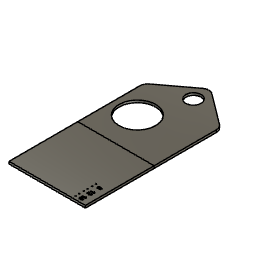
Lid (Autodesk Fusion 360 design; units mm, degrees)
Autodesk Fusion 360 part; units mm, degrees
sketch "Sketch1" plane through (0, 0, 0) normal (0, 0, 1) x (1, 0, 0)
  line L0 (0, 0) -> (100, 0)
  line L1 (100, 0) -> (100, 171.5)
  line L2 (100, 171.5) -> (0, 171.5)
  line L3 (0, 171.5) -> (0, 0)
  line L4 (56, 209.5) -> (96, 179.5)
  line L5 (4, 179.5) -> (44, 209.5)
  arc A0 (56, 209.5) -> (44, 209.5) centre (50, 201.5) ccw
  arc A1 (100, 171.5) -> (96, 179.5) centre (90, 171.5) ccw
  arc A2 (4, 179.5) -> (0, 171.5) centre (10, 171.5) ccw
  circle A3 centre (50, 191.5) radius 10
  dimension "d1" = 100
  dimension "d2" = 171.5
  dimension "d3" = 20
  dimension "d4" = 20
  dimension "d5" = 20
  dimension "d6" = 30
  dimension "d7" = 50
  dimension "d8" = 50
  dimension "d9" = 50
  dimension "d10" = 20
  dimension "d11" = 20
  dimension "d12" = 50
  constraint horizontal L0
  constraint vertical L1
  constraint horizontal L2
  constraint vertical L3
  constraint coincident L0.start L3.end
  constraint coincident L2 A2.centre
  constraint coincident L2 A1.centre
  constraint tangent L4 A1
  constraint tangent L5 A0
  measures "d1" distance of L0.start L0.end
  measures "d2" distance of L0.start L2.end
  measures "d3" diameter of A2
  measures "d4" diameter of A1
  measures "d5" diameter of A0
  measures "d6" distance of L2 A0.centre
  measures "d7" distance of L3 A0.centre
  measures "d8" distance of L5.start L5.end
  measures "d9" distance of L4.start L4.end
  measures "d10" diameter of A3
  measures "d11" distance of L2 A3.centre
  measures "d12" horizontal distance of L2.end A3.centre
extrude "Extrude1" add sketch "Sketch1" along normal blind 3 makes body 1
sketch "Sketch2" plane through (0, 0, 3) normal (0, 0, 1) x (-1, 0, 0)
  circle A0 centre (-50, -191.5) radius 10
  arc A1 (-56, -209.5) -> (-44, -209.5) centre (-50, -201.5) ccw
  line L0 (-44, -209.5) -> (-4, -179.5)
  arc A2 (-4, -179.5) -> (0, -171.5) centre (-10, -171.5) ccw
  line L1 (0, -171.5) -> (0, 0)
  line L2 (0, 0) -> (-100, 0)
  line L3 (-100, 0) -> (-100, -171.5)
  arc A3 (-100, -171.5) -> (-96, -179.5) centre (-90, -171.5) ccw
  line L4 (-96, -179.5) -> (-56, -209.5)
  line L5 (0, 0) -> (-100, 0) construction
  line L6 (-100, 0) -> (-100, -171.5) construction
  line L7 (-100, -171.5) -> (0, -171.5) construction
  line L8 (0, -171.5) -> (0, 0) construction
  circle A4 centre (-31.5, -136.5) radius 24
  dimension "d15" = 171.5
  dimension "d16" = 100
  dimension "d17" = 48
  dimension "d18" = 31.5
  dimension "d19" = 35
  constraint horizontal L5
  constraint vertical L6
  constraint horizontal L7
  constraint vertical L8
  constraint coincident L1.end L2.start
  measures "d15" distance of L1.end A2.end
  measures "d16" distance of L1.end L2.end
  measures "d17" diameter of A4
  measures "d18" distance of L8 A4.centre
  measures "d19" distance of L7 A4.centre
extrude "Extrude2" cut sketch "Sketch2" against normal blind 3 contours A4 bodies 1
sketch "Sketch3" plane through (0, 0, 3) normal (0, 0, 1) x (-1, 0, 0)
  circle A0 centre (-31.5, -136.5) radius 24
  circle A1 centre (-50, -191.5) radius 10
  arc A2 (-56, -209.5) -> (-44, -209.5) centre (-50, -201.5) ccw
  line L0 (-44, -209.5) -> (-4, -179.5)
  arc A3 (-4, -179.5) -> (0, -171.5) centre (-10, -171.5) ccw
  line L1 (0, -171.5) -> (0, 0)
  line L2 (0, 0) -> (-100, 0)
  line L3 (-100, 0) -> (-100, -171.5)
  arc A4 (-100, -171.5) -> (-96, -179.5) centre (-90, -171.5) ccw
  line L4 (-96, -179.5) -> (-56, -209.5)
  line L5 (-95, -65) -> (-95, 0) construction
  line L6 (-82, -5) -> (-83, -5)
  line L7 (-83, -5) -> (-83, -4)
  line L8 (-83, -4) -> (-82, -4)
  line L9 (-82, -4) -> (-82, -5)
  line L10 (-82, -10) -> (-83, -10)
  line L11 (-83, -10) -> (-83, -9)
  line L12 (-83, -9) -> (-82, -9)
  line L13 (-82, -9) -> (-82, -10)
  line L14 (-82, -16) -> (-83, -16)
  line L15 (-83, -16) -> (-83, -15)
  line L16 (-83, -15) -> (-82, -15)
  line L17 (-82, -15) -> (-82, -16)
  line L18 (-82, -21) -> (-83, -21)
  line L19 (-83, -21) -> (-83, -20)
  line L20 (-83, -20) -> (-82, -20)
  line L21 (-82, -20) -> (-82, -21)
  line L22 (-82, -27) -> (-83, -27)
  line L23 (-83, -27) -> (-83, -26)
  line L24 (-83, -26) -> (-82, -26)
  line L25 (-82, -26) -> (-82, -27)
  line L26 (-82, -32) -> (-83, -32)
  line L27 (-83, -32) -> (-83, -31)
  line L28 (-83, -31) -> (-82, -31)
  line L29 (-82, -31) -> (-82, -32)
  line L30 (-86, -35) -> (-86, 0) construction
  line L31 (-87, -32) -> (-87, -26) construction
  line L32 (-87, -26) -> (-92, -26) construction
  line L33 (-92, -26) -> (-92, -32) construction
  line L34 (-92, -32) -> (-87, -32) construction
  line L35 (-87, -21) -> (-87, -15) construction
  line L36 (-87, -15) -> (-92, -15) construction
  line L37 (-92, -15) -> (-92, -21) construction
  line L38 (-92, -21) -> (-87, -21) construction
  line L39 (-87, -10) -> (-87, -4) construction
  line L40 (-87, -4) -> (-92, -4) construction
  line L41 (-92, -4) -> (-92, -10) construction
  line L42 (-92, -10) -> (-87, -10) construction
  dimension "d22" = 5
  dimension "d23" = 1
  dimension "d24" = 1
  dimension "d25" = 1
  dimension "d26" = 1
  dimension "d27" = 1
  dimension "d28" = 1
  dimension "d29" = 1
  dimension "d30" = 1
  dimension "d31" = 1
  dimension "d32" = 1
  dimension "d33" = 1
  dimension "d34" = 1
  dimension "d36" = 5
  dimension "d37" = 6
  dimension "d38" = 6
  dimension "d39" = 5
  dimension "d40" = 6
  dimension "d41" = 5
  dimension "d42" = 5
  dimension "d43" = 5
  text T0 "8" font "Arial" height 5 bold align centre middle in box 6 x 5 at (-87, -32) x (0, 1) y (-1, 0) spacing 1 kerned
  text T1 "12" font "Arial" height 5 bold align centre middle in box 6 x 5 at (-87, -21) x (0, 1) y (-1, 0) spacing 1 kerned
  text T2 "16" font "Arial" height 5 bold align centre middle in box 6 x 5 at (-87, -10) x (0, 1) y (-1, 0) spacing 1 kerned
  constraint coincident L2 L5.end
  constraint perpendicular L2 L5
  constraint horizontal L6
  constraint vertical L7
  constraint horizontal L8
  constraint vertical L9
  constraint horizontal L10
  constraint vertical L11
  constraint horizontal L12
  constraint vertical L13
  constraint horizontal L14
  constraint vertical L15
  constraint horizontal L16
  constraint vertical L17
  constraint horizontal L18
  constraint vertical L19
  constraint horizontal L20
  constraint vertical L21
  constraint horizontal L22
  constraint vertical L23
  constraint horizontal L24
  constraint vertical L25
  constraint horizontal L26
  constraint vertical L27
  constraint horizontal L28
  constraint vertical L29
  constraint coincident L2 L30.end
  constraint perpendicular L2 L30
  measures "d22" distance of L3 L5
  measures "d23" distance of L10.end L11.end
  measures "d24" distance of L6.end L7.end
  measures "d25" distance of L14.end L15.end
  measures "d26" distance of L18.end L19.end
  measures "d27" distance of L22.end L23.end
  measures "d28" distance of L26.end L27.end
  measures "d29" distance of L26.start L26.end
  measures "d30" distance of L22.start L22.end
  measures "d31" distance of L18.start L18.end
  measures "d32" distance of L14.start L14.end
  measures "d33" distance of L10.start L10.end
  measures "d34" distance of L6.start L6.end
  measures "d36" distance of L18 L24
  measures "d37" distance of L24 L26
  measures "d38" distance of L16 L18
  measures "d39" distance of L10 L16
  measures "d40" distance of L8 L10
extrude "Extrude3" cut sketch "Sketch3" against normal blind 2 text T0 T1 T2 bodies 1
extrude "Extrude4" cut sketch "Sketch3" against normal blind 3 contours L6 L7 L8 L9 | L10 L11 L12 L13 | L14 L15 L16 L17 | L18 L19 L20 L21 | L22 L23 L24 L25 | L26 L27 L28 L29 bodies 1
sketch "Sketch4" plane through (0, 0, 3) normal (0, 0, 1) x (-1, 0, 0)
  line L0 (-83, -16) -> (-83, -15)
  line L1 (-83, -15) -> (-82, -15)
  line L2 (-82, -15) -> (-82, -16)
  line L3 (-82, -16) -> (-83, -16)
  line L4 (-83, -32) -> (-83, -31)
  line L5 (-83, -31) -> (-82, -31)
  line L6 (-82, -31) -> (-82, -32)
  line L7 (-82, -32) -> (-83, -32)
  line L8 (-83, -10) -> (-83, -9)
  line L9 (-83, -9) -> (-82, -9)
  line L10 (-82, -9) -> (-82, -10)
  line L11 (-82, -10) -> (-83, -10)
  line L12 (-83, -21) -> (-83, -20)
  line L13 (-83, -20) -> (-82, -20)
  line L14 (-82, -20) -> (-82, -21)
  line L15 (-82, -21) -> (-83, -21)
  line L16 (-83, -27) -> (-83, -26)
  line L17 (-83, -26) -> (-82, -26)
  line L18 (-82, -26) -> (-82, -27)
  line L19 (-82, -27) -> (-83, -27)
  line L20 (-83, -5) -> (-83, -4)
  line L21 (-83, -4) -> (-82, -4)
  line L22 (-82, -4) -> (-82, -5)
  line L23 (-82, -5) -> (-83, -5)
  arc A0 (-56, -209.5) -> (-44, -209.5) centre (-50, -201.5) ccw
  line L24 (-44, -209.5) -> (-4, -179.5)
  arc A1 (-4, -179.5) -> (0, -171.5) centre (-10, -171.5) ccw
  line L25 (0, -171.5) -> (0, 0)
  line L26 (0, 0) -> (-100, 0)
  line L27 (-100, 0) -> (-100, -171.5)
  arc A2 (-100, -171.5) -> (-96, -179.5) centre (-90, -171.5) ccw
  line L28 (-96, -179.5) -> (-56, -209.5)
  circle A3 centre (-50, -191.5) radius 10
  circle A4 centre (-31.5, -136.5) radius 24
  line L29 (-92.0205, -9.0651) -> (-92.0205, -8.2875)
  line L30 (-92.0205, -8.2875) -> (-87, -8.2875)
  line L31 (-87, -8.2875) -> (-87, -9.2459)
  line L32 (-87, -9.2459) -> (-90.6119, -9.2459)
  spline S0 degree 3 poles (-90.6119, -9.2459) (-90.4584, -9.4301) (-90.148, -9.8026) (-89.9736, -10.2552) (-89.8854, -10.484) knots 0 0 0 0 0.071402 0.144411 0.144411 0.144411 0.144411
  line L33 (-89.8854, -10.484) -> (-90.7551, -10.484)
  spline S1 degree 3 poles (-90.7551, -10.484) (-90.8095, -10.3508) (-90.9288, -10.0589) (-91.1179, -9.8062) (-91.2207, -9.6688) knots 0 0 0 0 0.042986 0.09421 0.09421 0.09421 0.09421
  spline S2 degree 3 poles (-91.2207, -9.6688) (-91.3367, -9.5348) (-91.5605, -9.2762) (-91.8709, -9.1338) (-92.0205, -9.0651) knots 0 0 0 0 0.052484 0.101245 0.101245 0.101245 0.101245
  line L34 (-92.0205, -20.014) -> (-92.0205, -19.2364)
  line L35 (-92.0205, -19.2364) -> (-87, -19.2364)
  line L36 (-87, -19.2364) -> (-87, -20.1947)
  line L37 (-87, -20.1947) -> (-90.6119, -20.1947)
  spline S3 degree 3 poles (-90.6119, -20.1947) (-90.4584, -20.3789) (-90.148, -20.7515) (-89.9736, -21.204) (-89.8854, -21.4328) knots 0 0 0 0 0.071402 0.144411 0.144411 0.144411 0.144411
  line L38 (-89.8854, -21.4328) -> (-90.7551, -21.4328)
  spline S4 degree 3 poles (-90.7551, -21.4328) (-90.8095, -21.2996) (-90.9288, -21.0078) (-91.1179, -20.7551) (-91.2207, -20.6177) knots 0 0 0 0 0.042986 0.09421 0.09421 0.09421 0.09421
  spline S5 degree 3 poles (-91.2207, -20.6177) (-91.3367, -20.4836) (-91.5605, -20.2251) (-91.8709, -20.0826) (-92.0205, -20.014) knots 0 0 0 0 0.052484 0.101245 0.101245 0.101245 0.101245
  spline S6 degree 3 poles (-88.4291, -30.6439) (-88.5611, -30.6358) (-88.8234, -30.6197) (-89.0579, -30.5014) (-89.1743, -30.4427) knots 0 0 0 0 0.039248 0.077913 0.077913 0.077913 0.077913
  spline S7 degree 3 poles (-89.1743, -30.4427) (-89.2822, -30.3628) (-89.5089, -30.1951) (-89.6329, -29.9412) (-89.6978, -29.8083) knots 0 0 0 0 0.03969 0.083332 0.083332 0.083332 0.083332
  spline S8 degree 3 poles (-89.6978, -29.8083) (-89.752, -29.9218) (-89.8541, -30.1359) (-90.0413, -30.2808) (-90.1293, -30.3489) knots 0 0 0 0 0.037117 0.070026 0.070026 0.070026 0.070026
  spline S9 degree 3 poles (-90.1293, -30.3489) (-90.2232, -30.3982) (-90.4119, -30.497) (-90.6245, -30.5108) (-90.7312, -30.5177) knots 0 0 0 0 0.03144 0.063142 0.063142 0.063142 0.063142
  spline S10 degree 3 poles (-90.7312, -30.5177) (-90.9088, -30.5023) (-91.2593, -30.4719) (-91.5246, -30.2411) (-91.6555, -30.1272) knots 0 0 0 0 0.051999 0.102674 0.102674 0.102674 0.102674
  spline S11 degree 3 poles (-91.6555, -30.1272) (-91.7618, -29.9748) (-91.9933, -29.6428) (-92.0109, -29.2367) (-92.0205, -29.0171) knots 0 0 0 0 0.054631 0.119017 0.119017 0.119017 0.119017
  spline S12 degree 3 poles (-92.0205, -29.0171) (-92.0106, -28.7989) (-91.9923, -28.3942) (-91.7618, -28.063) (-91.6555, -27.9103) knots 0 0 0 0 0.063964 0.118669 0.118669 0.118669 0.118669
  spline S13 degree 3 poles (-91.6555, -27.9103) (-91.5247, -27.7954) (-91.26, -27.5629) (-90.9089, -27.532) (-90.7312, -27.5164) knots 0 0 0 0 0.050824 0.102839 0.102839 0.102839 0.102839
  spline S14 degree 3 poles (-90.7312, -27.5164) (-90.6193, -27.5234) (-90.3992, -27.5371) (-90.2068, -27.6444) (-90.1122, -27.6971) knots 0 0 0 0 0.033179 0.065222 0.065222 0.065222 0.065222
  spline S15 degree 3 poles (-90.1122, -27.6971) (-90.0266, -27.7648) (-89.8511, -27.9035) (-89.7497, -28.1031) (-89.6978, -28.2053) knots 0 0 0 0 0.032323 0.06627 0.06627 0.06627 0.06627
  spline S16 degree 3 poles (-89.6978, -28.2053) (-89.638, -28.0765) (-89.5228, -27.8286) (-89.3116, -27.6557) (-89.2101, -27.5726) knots 0 0 0 0 0.041993 0.080807 0.080807 0.080807 0.080807
  spline S17 degree 3 poles (-89.2101, -27.5726) (-89.0977, -27.5095) (-88.8678, -27.3804) (-88.6045, -27.3643) (-88.47, -27.3561) knots 0 0 0 0 0.038162 0.07801 0.07801 0.07801 0.07801
  spline S18 degree 3 poles (-88.47, -27.3561) (-88.2525, -27.372) (-87.8308, -27.403) (-87.5031, -27.669) (-87.3445, -27.7977) knots 0 0 0 0 0.06372 0.123527 0.123527 0.123527 0.123527
  spline S19 degree 3 poles (-87.3445, -27.7977) (-87.2182, -27.9625) (-86.9531, -28.3083) (-86.9257, -28.7443) (-86.9113, -28.9727) knots 0 0 0 0 0.060855 0.127775 0.127775 0.127775 0.127775
  spline S20 degree 3 poles (-86.9113, -28.9727) (-86.9234, -29.1868) (-86.9464, -29.5966) (-87.165, -29.943) (-87.2694, -30.1085) knots 0 0 0 0 0.063138 0.120844 0.120844 0.120844 0.120844
  spline S21 degree 3 poles (-87.2694, -30.1085) (-87.4261, -30.2646) (-87.7466, -30.5841) (-88.1982, -30.6237) (-88.4291, -30.6439) knots 0 0 0 0 0.064238 0.131411 0.131411 0.131411 0.131411
  spline S22 degree 3 poles (-88.1562, -16.2742) (-88.1122, -16.312) (-88.0283, -16.3839) (-87.9347, -16.4425) (-87.8902, -16.4703) knots 0 0 0 0 0.017365 0.033092 0.033092 0.033092 0.033092
  line L39 (-87.8902, -16.4703) -> (-87.8902, -14.5672)
  line L40 (-87.8902, -14.5672) -> (-87, -14.5672)
  line L41 (-87, -14.5672) -> (-87, -17.9267)
  spline S23 degree 3 poles (-87, -17.9267) (-87.1668, -17.8989) (-87.5038, -17.8429) (-87.8047, -17.681) (-87.9567, -17.5992) knots 0 0 0 0 0.050353 0.101733 0.101733 0.101733 0.101733
  spline S24 degree 3 poles (-87.9567, -17.5992) (-88.1357, -17.4683) (-88.5712, -17.1498) (-88.939, -16.7543) (-89.1555, -16.5215) knots 0 0 0 0 0.066412 0.161523 0.161523 0.161523 0.161523
  spline S25 degree 3 poles (-89.1555, -16.5215) (-89.3199, -16.3425) (-89.5777, -16.0618) (-89.8686, -15.8159) (-89.9741, -15.7268) knots 0 0 0 0 0.072782 0.114179 0.114179 0.114179 0.114179
  spline S26 degree 3 poles (-89.9741, -15.7268) (-90.0697, -15.6692) (-90.2511, -15.5599) (-90.4614, -15.5389) (-90.5607, -15.529) knots 0 0 0 0 0.033023 0.0626 0.0626 0.0626 0.0626
  spline S27 degree 3 poles (-90.5607, -15.529) (-90.6588, -15.5337) (-90.8409, -15.5424) (-90.9864, -15.6511) (-91.0535, -15.7012) knots 0 0 0 0 0.028676 0.053274 0.053274 0.053274 0.053274
  spline S28 degree 3 poles (-91.0535, -15.7012) (-91.1037, -15.7669) (-91.2107, -15.9069) (-91.2205, -16.0833) (-91.2258, -16.177) knots 0 0 0 0 0.024236 0.051648 0.051648 0.051648 0.051648
  spline S29 degree 3 poles (-91.2258, -16.177) (-91.2198, -16.2704) (-91.2084, -16.4486) (-91.0977, -16.5881) (-91.045, -16.6545) knots 0 0 0 0 0.02732 0.052153 0.052153 0.052153 0.052153
  spline S30 degree 3 poles (-91.045, -16.6545) (-90.9673, -16.7076) (-90.7873, -16.8306) (-90.5688, -16.8488) (-90.4447, -16.8591) knots 0 0 0 0 0.027816 0.064377 0.064377 0.064377 0.064377
  line L42 (-90.4447, -16.8591) -> (-90.5402, -17.8141)
  spline S31 degree 3 poles (-90.5402, -17.8141) (-90.7784, -17.7788) (-91.2135, -17.7143) (-91.5319, -17.4144) (-91.676, -17.2786) knots 0 0 0 0 0.070212 0.128259 0.128259 0.128259 0.128259
  spline S32 degree 3 poles (-91.676, -17.2786) (-91.7764, -17.1143) (-91.9872, -16.7694) (-92.009, -16.3649) (-92.0205, -16.1531) knots 0 0 0 0 0.056857 0.119356 0.119356 0.119356 0.119356
  spline S33 degree 3 poles (-92.0205, -16.1531) (-92.0088, -15.9252) (-91.9868, -15.4977) (-91.7377, -15.1516) (-91.6214, -14.9901) knots 0 0 0 0 0.06683 0.125293 0.125293 0.125293 0.125293
  spline S34 degree 3 poles (-91.6214, -14.9901) (-91.4797, -14.8668) (-91.1947, -14.6186) (-90.8183, -14.5844) (-90.6289, -14.5672) knots 0 0 0 0 0.054863 0.110365 0.110365 0.110365 0.110365
  spline S35 degree 3 poles (-90.6289, -14.5672) (-90.5181, -14.5721) (-90.298, -14.5818) (-90.0895, -14.653) (-89.986, -14.6883) knots 0 0 0 0 0.033094 0.065719 0.065719 0.065719 0.065719
  spline S36 degree 3 poles (-89.986, -14.6883) (-89.8799, -14.7371) (-89.6528, -14.8415) (-89.4529, -14.9919) (-89.3465, -15.072) knots 0 0 0 0 0.034948 0.074768 0.074768 0.074768 0.074768
  spline S37 degree 3 poles (-89.3465, -15.072) (-89.2552, -15.152) (-89.0305, -15.3487) (-88.8286, -15.5689) (-88.7087, -15.6995) knots 0 0 0 0 0.036404 0.089534 0.089534 0.089534 0.089534
  spline S38 degree 3 poles (-88.7087, -15.6995) (-88.5948, -15.8245) (-88.4158, -16.021) (-88.2255, -16.2066) (-88.1562, -16.2742) knots 0 0 0 0 0.050705 0.079736 0.079736 0.079736 0.079736
  spline S39 degree 3 poles (-92.0205, -5.0269) (-92.0095, -4.848) (-91.9884, -4.5042) (-91.7945, -4.2201) (-91.7016, -4.0839) knots 0 0 0 0 0.052662 0.101211 0.101211 0.101211 0.101211
  spline S40 degree 3 poles (-91.7016, -4.0839) (-91.5777, -3.9699) (-91.3136, -3.7268) (-90.9621, -3.6493) (-90.7756, -3.6081) knots 0 0 0 0 0.049626 0.10577 0.10577 0.10577 0.10577
  line L43 (-90.7756, -3.6081) -> (-90.6733, -4.5358)
  spline S41 degree 3 poles (-90.6733, -4.5358) (-90.7595, -4.5489) (-90.9161, -4.5725) (-91.0404, -4.6696) (-91.0962, -4.7132) knots 0 0 0 0 0.025643 0.046549 0.046549 0.046549 0.046549
  spline S42 degree 3 poles (-91.0962, -4.7132) (-91.136, -4.7659) (-91.2188, -4.8757) (-91.2279, -5.0134) (-91.2326, -5.0849) knots 0 0 0 0 0.019378 0.040376 0.040376 0.040376 0.040376
  spline S43 degree 3 poles (-91.2326, -5.0849) (-91.2197, -5.1834) (-91.1928, -5.3878) (-91.0393, -5.5264) (-90.9598, -5.5982) knots 0 0 0 0 0.028828 0.059854 0.059854 0.059854 0.059854
  spline S44 degree 3 poles (-90.9598, -5.5982) (-90.8215, -5.6624) (-90.4636, -5.8287) (-90.0673, -5.8497) (-89.824, -5.8626) knots 0 0 0 0 0.04538 0.117524 0.117524 0.117524 0.117524
  spline S45 degree 3 poles (-89.824, -5.8626) (-89.9474, -5.737) (-90.1912, -5.4888) (-90.2285, -5.1432) (-90.2469, -4.9724) knots 0 0 0 0 0.051176 0.101164 0.101164 0.101164 0.101164
  spline S46 degree 3 poles (-90.2469, -4.9724) (-90.227, -4.7786) (-90.1866, -4.3864) (-89.9232, -4.0927) (-89.7899, -3.9441) knots 0 0 0 0 0.056881 0.115141 0.115141 0.115141 0.115141
  spline S47 degree 3 poles (-89.7899, -3.9441) (-89.622, -3.8193) (-89.2722, -3.5593) (-88.8364, -3.5308) (-88.6098, -3.516) knots 0 0 0 0 0.061412 0.127933 0.127933 0.127933 0.127933
  spline S48 degree 3 poles (-88.6098, -3.516) (-88.3708, -3.5309) (-87.9146, -3.5594) (-87.5515, -3.835) (-87.3786, -3.9662) knots 0 0 0 0 0.070061 0.133726 0.133726 0.133726 0.133726
  spline S49 degree 3 poles (-87.3786, -3.9662) (-87.2433, -4.1298) (-86.9659, -4.4651) (-86.9321, -4.8997) (-86.9147, -5.1224) knots 0 0 0 0 0.062079 0.127323 0.127323 0.127323 0.127323
  spline S50 degree 3 poles (-86.9147, -5.1224) (-86.9395, -5.3638) (-86.9892, -5.8479) (-87.3315, -6.1939) (-87.5031, -6.3673) knots 0 0 0 0 0.070531 0.141441 0.141441 0.141441 0.141441
  spline S51 degree 3 poles (-87.5031, -6.3673) (-87.7564, -6.5088) (-88.3517, -6.8413) (-89.0377, -6.85) (-89.4318, -6.855) knots 0 0 0 0 0.085821 0.201701 0.201701 0.201701 0.201701
  spline S52 degree 3 poles (-89.4318, -6.855) (-89.8364, -6.8495) (-90.5422, -6.8398) (-91.1528, -6.4943) (-91.4134, -6.3469) knots 0 0 0 0 0.118944 0.207464 0.207464 0.207464 0.207464
  spline S53 degree 3 poles (-91.4134, -6.3469) (-91.5904, -6.1639) (-91.9471, -5.7952) (-91.9959, -5.2843) (-92.0205, -5.0269) knots 0 0 0 0 0.074058 0.149191 0.149191 0.149191 0.149191
sketch "Sketch5" plane through (0, 0, 3) normal (0, 0, 1) x (-1, 0, 0)
  line L0 (-68, -32) -> (-67, -32)
  line L1 (-67, -32) -> (-67, -31)
  line L2 (-67, -31) -> (-68, -31)
  line L3 (-68, -31) -> (-68, -32)
  line L4 (-68, -27) -> (-67, -27)
  line L5 (-67, -27) -> (-67, -26)
  line L6 (-67, -26) -> (-68, -26)
  line L7 (-68, -26) -> (-68, -27)
  line L8 (-68, -21) -> (-67, -21)
  line L9 (-67, -21) -> (-67, -20)
  line L10 (-67, -20) -> (-68, -20)
  line L11 (-68, -20) -> (-68, -21)
  line L12 (-68, -16) -> (-67, -16)
  line L13 (-67, -16) -> (-67, -15)
  line L14 (-67, -15) -> (-68, -15)
  line L15 (-68, -15) -> (-68, -16)
  line L16 (-68, -10) -> (-67, -10)
  line L17 (-67, -10) -> (-67, -9)
  line L18 (-67, -9) -> (-68, -9)
  line L19 (-68, -9) -> (-68, -10)
  line L20 (-68, -5) -> (-67, -5)
  line L21 (-67, -5) -> (-67, -4)
  line L22 (-67, -4) -> (-68, -4)
  line L23 (-68, -4) -> (-68, -5)
  constraint horizontal L0
  constraint vertical L1
  constraint horizontal L2
  constraint vertical L3
  constraint horizontal L4
  constraint vertical L5
  constraint horizontal L6
  constraint vertical L7
  constraint horizontal L8
  constraint vertical L9
  constraint horizontal L10
  constraint vertical L11
  constraint horizontal L12
  constraint vertical L13
  constraint horizontal L14
  constraint vertical L15
  constraint horizontal L16
  constraint vertical L17
  constraint horizontal L18
  constraint vertical L19
  constraint horizontal L20
  constraint vertical L21
  constraint horizontal L22
  constraint vertical L23
extrude "Extrude5" cut sketch "Sketch5" against normal blind 3 bodies 1
sketch "Sketch6" plane through (0, 0, 3) normal (0, 0, 1) x (-1, 0, 0)
  line L0 (-71, -32) -> (-71, 0) construction
  line L1 (-72, -32) -> (-72, -26) construction
  line L2 (-72, -26) -> (-78, -26) construction
  line L3 (-78, -26) -> (-78, -32) construction
  line L4 (-78, -32) -> (-72, -32) construction
  line L5 (-72, -21) -> (-72, -15) construction
  line L6 (-72, -15) -> (-78, -15) construction
  line L7 (-78, -15) -> (-78, -21) construction
  line L8 (-78, -21) -> (-72, -21) construction
  line L9 (-72, -10) -> (-72, -4) construction
  line L10 (-72, -4) -> (-78, -4) construction
  line L11 (-78, -4) -> (-78, -10) construction
  line L12 (-78, -10) -> (-72, -10) construction
  dimension "d50" = 5
  dimension "d51" = 5
  dimension "d52" = 5
  text T0 "H" font "Arial" height 5 bold align centre middle in box 6 x 6 at (-72, -32) x (0, 1) y (-1, 0) spacing 1 kerned
  text T1 "M" font "Arial" height 5 bold align centre middle in box 6 x 6 at (-72, -21) x (0, 1) y (-1, 0) spacing 1 kerned
  text T2 "L" font "Arial" height 5 bold align centre middle in box 6 x 6 at (-72, -10) x (0, 1) y (-1, 0) spacing 1 kerned
  constraint vertical L0
extrude "Extrude6" cut sketch "Sketch6" against normal blind 2 text T0 T1 T2 bodies 1
ref_plane "WorkPlane1" through (0, 90, 0) normal (0, 1, 0) x (0, 0, 1)
split "Split1" by plane through (0, 90, 0) normal (0, 1, 0) bodies 1 makes body 2 at (85.0773, 131.4743, 0)
sketch "Sketch8" plane through (0, 0, 3) normal (0, 0, 1) x (-1, 0, 0)
  spline S0 degree 3 poles (-92.0205, -5.0269) (-92.0095, -4.848) (-91.9884, -4.5042) (-91.7945, -4.2201) (-91.7016, -4.0839) knots 0 0 0 0 0.052662 0.101211 0.101211 0.101211 0.101211
  spline S1 degree 3 poles (-91.7016, -4.0839) (-91.5777, -3.9699) (-91.3136, -3.7268) (-90.9621, -3.6493) (-90.7756, -3.6081) knots 0 0 0 0 0.049626 0.10577 0.10577 0.10577 0.10577
  line L0 (-90.7756, -3.6081) -> (-90.6733, -4.5358)
  spline S2 degree 3 poles (-90.6733, -4.5358) (-90.7595, -4.5489) (-90.9161, -4.5725) (-91.0404, -4.6696) (-91.0962, -4.7132) knots 0 0 0 0 0.025643 0.046549 0.046549 0.046549 0.046549
  spline S3 degree 3 poles (-91.0962, -4.7132) (-91.136, -4.7659) (-91.2188, -4.8757) (-91.2279, -5.0134) (-91.2326, -5.0849) knots 0 0 0 0 0.019378 0.040376 0.040376 0.040376 0.040376
  spline S4 degree 3 poles (-91.2326, -5.0849) (-91.2197, -5.1834) (-91.1928, -5.3878) (-91.0393, -5.5264) (-90.9598, -5.5982) knots 0 0 0 0 0.028828 0.059854 0.059854 0.059854 0.059854
  spline S5 degree 3 poles (-90.9598, -5.5982) (-90.8215, -5.6624) (-90.4636, -5.8287) (-90.0673, -5.8497) (-89.824, -5.8626) knots 0 0 0 0 0.04538 0.117524 0.117524 0.117524 0.117524
  spline S6 degree 3 poles (-89.824, -5.8626) (-89.9474, -5.737) (-90.1912, -5.4888) (-90.2285, -5.1432) (-90.2469, -4.9724) knots 0 0 0 0 0.051176 0.101164 0.101164 0.101164 0.101164
  spline S7 degree 3 poles (-90.2469, -4.9724) (-90.227, -4.7786) (-90.1866, -4.3864) (-89.9232, -4.0927) (-89.7899, -3.9441) knots 0 0 0 0 0.056881 0.115141 0.115141 0.115141 0.115141
  spline S8 degree 3 poles (-89.7899, -3.9441) (-89.622, -3.8193) (-89.2722, -3.5593) (-88.8364, -3.5308) (-88.6098, -3.516) knots 0 0 0 0 0.061412 0.127933 0.127933 0.127933 0.127933
  spline S9 degree 3 poles (-88.6098, -3.516) (-88.3708, -3.5309) (-87.9146, -3.5594) (-87.5515, -3.835) (-87.3786, -3.9662) knots 0 0 0 0 0.070061 0.133726 0.133726 0.133726 0.133726
  spline S10 degree 3 poles (-87.3786, -3.9662) (-87.2433, -4.1298) (-86.9659, -4.4651) (-86.9321, -4.8997) (-86.9147, -5.1224) knots 0 0 0 0 0.062079 0.127323 0.127323 0.127323 0.127323
  spline S11 degree 3 poles (-86.9147, -5.1224) (-86.9395, -5.3638) (-86.9892, -5.8479) (-87.3315, -6.1939) (-87.5031, -6.3673) knots 0 0 0 0 0.070531 0.141441 0.141441 0.141441 0.141441
  spline S12 degree 3 poles (-87.5031, -6.3673) (-87.7564, -6.5088) (-88.3517, -6.8413) (-89.0377, -6.85) (-89.4318, -6.855) knots 0 0 0 0 0.085821 0.201701 0.201701 0.201701 0.201701
  spline S13 degree 3 poles (-89.4318, -6.855) (-89.8364, -6.8495) (-90.5422, -6.8398) (-91.1528, -6.4943) (-91.4134, -6.3469) knots 0 0 0 0 0.118944 0.207464 0.207464 0.207464 0.207464
  spline S14 degree 3 poles (-91.4134, -6.3469) (-91.5904, -6.1639) (-91.9471, -5.7952) (-91.9959, -5.2843) (-92.0205, -5.0269) knots 0 0 0 0 0.074058 0.149191 0.149191 0.149191 0.149191
  spline S15 degree 3 poles (-88.1562, -16.2742) (-88.1122, -16.312) (-88.0283, -16.3839) (-87.9347, -16.4425) (-87.8902, -16.4703) knots 0 0 0 0 0.017365 0.033092 0.033092 0.033092 0.033092
  line L1 (-87.8902, -16.4703) -> (-87.8902, -14.5672)
  line L2 (-87.8902, -14.5672) -> (-87, -14.5672)
  line L3 (-87, -14.5672) -> (-87, -17.9267)
  spline S16 degree 3 poles (-87, -17.9267) (-87.1668, -17.8989) (-87.5038, -17.8429) (-87.8047, -17.681) (-87.9567, -17.5992) knots 0 0 0 0 0.050353 0.101733 0.101733 0.101733 0.101733
  spline S17 degree 3 poles (-87.9567, -17.5992) (-88.1357, -17.4683) (-88.5712, -17.1498) (-88.939, -16.7543) (-89.1555, -16.5215) knots 0 0 0 0 0.066412 0.161523 0.161523 0.161523 0.161523
  spline S18 degree 3 poles (-89.1555, -16.5215) (-89.3199, -16.3425) (-89.5777, -16.0618) (-89.8686, -15.8159) (-89.9741, -15.7268) knots 0 0 0 0 0.072782 0.114179 0.114179 0.114179 0.114179
  spline S19 degree 3 poles (-89.9741, -15.7268) (-90.0697, -15.6692) (-90.2511, -15.5599) (-90.4614, -15.5389) (-90.5607, -15.529) knots 0 0 0 0 0.033023 0.0626 0.0626 0.0626 0.0626
  spline S20 degree 3 poles (-90.5607, -15.529) (-90.6588, -15.5337) (-90.8409, -15.5424) (-90.9864, -15.6511) (-91.0535, -15.7012) knots 0 0 0 0 0.028676 0.053274 0.053274 0.053274 0.053274
  spline S21 degree 3 poles (-91.0535, -15.7012) (-91.1037, -15.7669) (-91.2107, -15.9069) (-91.2205, -16.0833) (-91.2258, -16.177) knots 0 0 0 0 0.024236 0.051648 0.051648 0.051648 0.051648
  spline S22 degree 3 poles (-91.2258, -16.177) (-91.2198, -16.2704) (-91.2084, -16.4486) (-91.0977, -16.5881) (-91.045, -16.6545) knots 0 0 0 0 0.02732 0.052153 0.052153 0.052153 0.052153
  spline S23 degree 3 poles (-91.045, -16.6545) (-90.9673, -16.7076) (-90.7873, -16.8306) (-90.5688, -16.8488) (-90.4447, -16.8591) knots 0 0 0 0 0.027816 0.064377 0.064377 0.064377 0.064377
  line L4 (-90.4447, -16.8591) -> (-90.5402, -17.8141)
  spline S24 degree 3 poles (-90.5402, -17.8141) (-90.7784, -17.7788) (-91.2135, -17.7143) (-91.5319, -17.4144) (-91.676, -17.2786) knots 0 0 0 0 0.070212 0.128259 0.128259 0.128259 0.128259
  spline S25 degree 3 poles (-91.676, -17.2786) (-91.7764, -17.1143) (-91.9872, -16.7694) (-92.009, -16.3649) (-92.0205, -16.1531) knots 0 0 0 0 0.056857 0.119356 0.119356 0.119356 0.119356
  spline S26 degree 3 poles (-92.0205, -16.1531) (-92.0088, -15.9252) (-91.9868, -15.4977) (-91.7377, -15.1516) (-91.6214, -14.9901) knots 0 0 0 0 0.06683 0.125293 0.125293 0.125293 0.125293
  spline S27 degree 3 poles (-91.6214, -14.9901) (-91.4797, -14.8668) (-91.1947, -14.6186) (-90.8183, -14.5844) (-90.6289, -14.5672) knots 0 0 0 0 0.054863 0.110365 0.110365 0.110365 0.110365
  spline S28 degree 3 poles (-90.6289, -14.5672) (-90.5181, -14.5721) (-90.298, -14.5818) (-90.0895, -14.653) (-89.986, -14.6883) knots 0 0 0 0 0.033094 0.065719 0.065719 0.065719 0.065719
  spline S29 degree 3 poles (-89.986, -14.6883) (-89.8799, -14.7371) (-89.6528, -14.8415) (-89.4529, -14.9919) (-89.3465, -15.072) knots 0 0 0 0 0.034948 0.074768 0.074768 0.074768 0.074768
  spline S30 degree 3 poles (-89.3465, -15.072) (-89.2552, -15.152) (-89.0305, -15.3487) (-88.8286, -15.5689) (-88.7087, -15.6995) knots 0 0 0 0 0.036404 0.089534 0.089534 0.089534 0.089534
  spline S31 degree 3 poles (-88.7087, -15.6995) (-88.5948, -15.8245) (-88.4158, -16.021) (-88.2255, -16.2066) (-88.1562, -16.2742) knots 0 0 0 0 0.050705 0.079736 0.079736 0.079736 0.079736
  spline S32 degree 3 poles (-88.4291, -30.6439) (-88.5611, -30.6358) (-88.8234, -30.6197) (-89.0579, -30.5014) (-89.1743, -30.4427) knots 0 0 0 0 0.039248 0.077913 0.077913 0.077913 0.077913
  spline S33 degree 3 poles (-89.1743, -30.4427) (-89.2822, -30.3628) (-89.5089, -30.1951) (-89.6329, -29.9412) (-89.6978, -29.8083) knots 0 0 0 0 0.03969 0.083332 0.083332 0.083332 0.083332
  spline S34 degree 3 poles (-89.6978, -29.8083) (-89.752, -29.9218) (-89.8541, -30.1359) (-90.0413, -30.2808) (-90.1293, -30.3489) knots 0 0 0 0 0.037117 0.070026 0.070026 0.070026 0.070026
  spline S35 degree 3 poles (-90.1293, -30.3489) (-90.2232, -30.3982) (-90.4119, -30.497) (-90.6245, -30.5108) (-90.7312, -30.5177) knots 0 0 0 0 0.03144 0.063142 0.063142 0.063142 0.063142
  spline S36 degree 3 poles (-90.7312, -30.5177) (-90.9088, -30.5023) (-91.2593, -30.4719) (-91.5246, -30.2411) (-91.6555, -30.1272) knots 0 0 0 0 0.051999 0.102674 0.102674 0.102674 0.102674
  spline S37 degree 3 poles (-91.6555, -30.1272) (-91.7618, -29.9748) (-91.9933, -29.6428) (-92.0109, -29.2367) (-92.0205, -29.0171) knots 0 0 0 0 0.054631 0.119017 0.119017 0.119017 0.119017
  spline S38 degree 3 poles (-92.0205, -29.0171) (-92.0106, -28.7989) (-91.9923, -28.3942) (-91.7618, -28.063) (-91.6555, -27.9103) knots 0 0 0 0 0.063964 0.118669 0.118669 0.118669 0.118669
  spline S39 degree 3 poles (-91.6555, -27.9103) (-91.5247, -27.7954) (-91.26, -27.5629) (-90.9089, -27.532) (-90.7312, -27.5164) knots 0 0 0 0 0.050824 0.102839 0.102839 0.102839 0.102839
  spline S40 degree 3 poles (-90.7312, -27.5164) (-90.6193, -27.5234) (-90.3992, -27.5371) (-90.2068, -27.6444) (-90.1122, -27.6971) knots 0 0 0 0 0.033179 0.065222 0.065222 0.065222 0.065222
  spline S41 degree 3 poles (-90.1122, -27.6971) (-90.0266, -27.7648) (-89.8511, -27.9035) (-89.7497, -28.1031) (-89.6978, -28.2053) knots 0 0 0 0 0.032323 0.06627 0.06627 0.06627 0.06627
  spline S42 degree 3 poles (-89.6978, -28.2053) (-89.638, -28.0765) (-89.5228, -27.8286) (-89.3116, -27.6557) (-89.2101, -27.5726) knots 0 0 0 0 0.041993 0.080807 0.080807 0.080807 0.080807
  spline S43 degree 3 poles (-89.2101, -27.5726) (-89.0977, -27.5095) (-88.8678, -27.3804) (-88.6045, -27.3643) (-88.47, -27.3561) knots 0 0 0 0 0.038162 0.07801 0.07801 0.07801 0.07801
  spline S44 degree 3 poles (-88.47, -27.3561) (-88.2525, -27.372) (-87.8308, -27.403) (-87.5031, -27.669) (-87.3445, -27.7977) knots 0 0 0 0 0.06372 0.123527 0.123527 0.123527 0.123527
  spline S45 degree 3 poles (-87.3445, -27.7977) (-87.2182, -27.9625) (-86.9531, -28.3083) (-86.9257, -28.7443) (-86.9113, -28.9727) knots 0 0 0 0 0.060855 0.127775 0.127775 0.127775 0.127775
  spline S46 degree 3 poles (-86.9113, -28.9727) (-86.9234, -29.1868) (-86.9464, -29.5966) (-87.165, -29.943) (-87.2694, -30.1085) knots 0 0 0 0 0.063138 0.120844 0.120844 0.120844 0.120844
  spline S47 degree 3 poles (-87.2694, -30.1085) (-87.4261, -30.2646) (-87.7466, -30.5841) (-88.1982, -30.6237) (-88.4291, -30.6439) knots 0 0 0 0 0.064238 0.131411 0.131411 0.131411 0.131411
  line L5 (-92.0205, -20.014) -> (-92.0205, -19.2364)
  line L6 (-92.0205, -19.2364) -> (-87, -19.2364)
  line L7 (-87, -19.2364) -> (-87, -20.1947)
  line L8 (-87, -20.1947) -> (-90.6119, -20.1947)
  spline S48 degree 3 poles (-90.6119, -20.1947) (-90.4584, -20.3789) (-90.148, -20.7515) (-89.9736, -21.204) (-89.8854, -21.4328) knots 0 0 0 0 0.071402 0.144411 0.144411 0.144411 0.144411
  line L9 (-89.8854, -21.4328) -> (-90.7551, -21.4328)
  spline S49 degree 3 poles (-90.7551, -21.4328) (-90.8095, -21.2996) (-90.9288, -21.0078) (-91.1179, -20.7551) (-91.2207, -20.6177) knots 0 0 0 0 0.042986 0.09421 0.09421 0.09421 0.09421
  spline S50 degree 3 poles (-91.2207, -20.6177) (-91.3367, -20.4836) (-91.5605, -20.2251) (-91.8709, -20.0826) (-92.0205, -20.014) knots 0 0 0 0 0.052484 0.101245 0.101245 0.101245 0.101245
  line L10 (-92.0205, -9.0651) -> (-92.0205, -8.2875)
  line L11 (-92.0205, -8.2875) -> (-87, -8.2875)
  line L12 (-87, -8.2875) -> (-87, -9.2459)
  line L13 (-87, -9.2459) -> (-90.6119, -9.2459)
  spline S51 degree 3 poles (-90.6119, -9.2459) (-90.4584, -9.4301) (-90.148, -9.8026) (-89.9736, -10.2552) (-89.8854, -10.484) knots 0 0 0 0 0.071402 0.144411 0.144411 0.144411 0.144411
  line L14 (-89.8854, -10.484) -> (-90.7551, -10.484)
  spline S52 degree 3 poles (-90.7551, -10.484) (-90.8095, -10.3508) (-90.9288, -10.0589) (-91.1179, -9.8062) (-91.2207, -9.6688) knots 0 0 0 0 0.042986 0.09421 0.09421 0.09421 0.09421
  spline S53 degree 3 poles (-91.2207, -9.6688) (-91.3367, -9.5348) (-91.5605, -9.2762) (-91.8709, -9.1338) (-92.0205, -9.0651) knots 0 0 0 0 0.052484 0.101245 0.101245 0.101245 0.101245
  line L15 (-100, -90) -> (0, -90)
  line L16 (0, -90) -> (0, 0)
  line L17 (0, 0) -> (-100, 0)
  line L18 (-100, 0) -> (-100, -90)
  line L19 (-83, -5) -> (-83, -4)
  line L20 (-83, -4) -> (-82, -4)
  line L21 (-82, -4) -> (-82, -5)
  line L22 (-82, -5) -> (-83, -5)
  line L23 (-83, -27) -> (-83, -26)
  line L24 (-83, -26) -> (-82, -26)
  line L25 (-82, -26) -> (-82, -27)
  line L26 (-82, -27) -> (-83, -27)
  line L27 (-83, -21) -> (-83, -20)
  line L28 (-83, -20) -> (-82, -20)
  line L29 (-82, -20) -> (-82, -21)
  line L30 (-82, -21) -> (-83, -21)
  line L31 (-83, -10) -> (-83, -9)
  line L32 (-83, -9) -> (-82, -9)
  line L33 (-82, -9) -> (-82, -10)
  line L34 (-82, -10) -> (-83, -10)
  line L35 (-83, -32) -> (-83, -31)
  line L36 (-83, -31) -> (-82, -31)
  line L37 (-82, -31) -> (-82, -32)
  line L38 (-82, -32) -> (-83, -32)
  line L39 (-83, -16) -> (-83, -15)
  line L40 (-83, -15) -> (-82, -15)
  line L41 (-82, -15) -> (-82, -16)
  line L42 (-82, -16) -> (-83, -16)
  line L43 (-67, -32) -> (-68, -32)
  line L44 (-68, -32) -> (-68, -31)
  line L45 (-68, -31) -> (-67, -31)
  line L46 (-67, -31) -> (-67, -32)
  line L47 (-67, -10) -> (-68, -10)
  line L48 (-68, -10) -> (-68, -9)
  line L49 (-68, -9) -> (-67, -9)
  line L50 (-67, -9) -> (-67, -10)
  line L51 (-67, -16) -> (-68, -16)
  line L52 (-68, -16) -> (-68, -15)
  line L53 (-68, -15) -> (-67, -15)
  line L54 (-67, -15) -> (-67, -16)
  line L55 (-67, -27) -> (-68, -27)
  line L56 (-68, -27) -> (-68, -26)
  line L57 (-68, -26) -> (-67, -26)
  line L58 (-67, -26) -> (-67, -27)
  line L59 (-67, -5) -> (-68, -5)
  line L60 (-68, -5) -> (-68, -4)
  line L61 (-68, -4) -> (-67, -4)
  line L62 (-67, -4) -> (-67, -5)
  line L63 (-67, -21) -> (-68, -21)
  line L64 (-68, -21) -> (-68, -20)
  line L65 (-68, -20) -> (-67, -20)
  line L66 (-67, -20) -> (-67, -21)
  line L67 (-73.3629, -5.2401) -> (-72.5205, -5.2401)
  line L68 (-72.5205, -5.2401) -> (-72.5205, -8.7599)
  line L69 (-72.5205, -8.7599) -> (-77.4795, -8.7599)
  line L70 (-77.4795, -8.7599) -> (-77.4795, -7.7503)
  line L71 (-77.4795, -7.7503) -> (-73.3629, -7.7503)
  line L72 (-73.3629, -7.7503) -> (-73.3629, -5.2401)
  line L73 (-74.6862, -29.9891) -> (-72.5, -29.9891)
  line L74 (-72.5, -29.9891) -> (-72.5, -30.9986)
  line L75 (-72.5, -30.9986) -> (-77.5, -30.9986)
  line L76 (-77.5, -30.9986) -> (-77.5, -29.9891)
  line L77 (-77.5, -29.9891) -> (-75.5321, -29.9891)
  line L78 (-75.5321, -29.9891) -> (-75.5321, -28.0109)
  line L79 (-75.5321, -28.0109) -> (-77.5, -28.0109)
  line L80 (-77.5, -28.0109) -> (-77.5, -27.0014)
  line L81 (-77.5, -27.0014) -> (-72.5, -27.0014)
  line L82 (-72.5, -27.0014) -> (-72.5, -28.0109)
  line L83 (-72.5, -28.0109) -> (-74.6862, -28.0109)
  line L84 (-74.6862, -28.0109) -> (-74.6862, -29.9891)
  line L85 (-76.4359, -19.4768) -> (-72.5, -19.4768)
  line L86 (-72.5, -19.4768) -> (-72.5, -20.4147)
  line L87 (-72.5, -20.4147) -> (-77.5, -20.4147)
  line L88 (-77.5, -20.4147) -> (-77.5, -18.9038)
  line L89 (-77.5, -18.9038) -> (-74.0894, -17.9966)
  line L90 (-74.0894, -17.9966) -> (-77.5, -17.0996)
  line L91 (-77.5, -17.0996) -> (-77.5, -15.5853)
  line L92 (-77.5, -15.5853) -> (-72.5, -15.5853)
  line L93 (-72.5, -15.5853) -> (-72.5, -16.5232)
  line L94 (-72.5, -16.5232) -> (-76.4359, -16.5232)
  line L95 (-76.4359, -16.5232) -> (-72.5, -17.5157)
  line L96 (-72.5, -17.5157) -> (-72.5, -18.4877)
  line L97 (-72.5, -18.4877) -> (-76.4359, -19.4768)
  line L98 (-80, 0) -> (-63, 0)
  line L99 (-63, 0) -> (-63, -33)
  line L100 (-63, -33) -> (-80, -33)
  line L101 (-80, -33) -> (-80, 0)
  constraint horizontal L98
  constraint vertical L99
  constraint horizontal L100
  constraint vertical L101
  constraint coincident L17 L98.start
extrude "Extrude8" add sketch "Sketch8" 1 faces at (85.0773, 131.4743, 3) against normal blind 3 contours L43 L44 L45 L46 | L47 L48 L49 L50 | L51 L52 L53 L54 | L55 L56 L57 L58 | L59 L60 L61 L62 | L63 L64 L65 L66 | L67 L68 L69 L70 L71 L72 | L73 L74 L75 L76 L77 L78 L79 L80 L81 L82 L83 L84 | L85 L86 L87 L88 L89 L90 L91 L92 L93 L94 L95 L96 L97 on bodies 2 bodies 1 2
split "Split2" by plane through (0, 90, 0) normal (0, 1, 0) bodies 1 makes body 3 at (85.0773, 131.4743, 0)
delete_body "RemoveBody1" bodies 2
sketch "Sketch7" plane through (0, 0, 3) normal (0, 0, 1) x (-1, 0, 0)
  line L0 (-100, 0) -> (0, 0)
  line L1 (0, 0) -> (0, -90)
  line L2 (0, -90) -> (-100, -90)
  line L3 (-100, -90) -> (-100, 0)
  constraint horizontal L0
  constraint vertical L1
  constraint horizontal L2
  constraint vertical L3
extrude "Extrude7" [suppressed]
